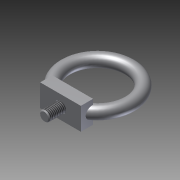
# Autodesk Inventor part: May Tec 1.71.30365_Installation ring_36.5
Saved by Autodesk Inventor 2011 SP1 (Build 150282100, 282)
## iProperties
Created: 2012-12-06
Part Number: May Tec 1.71.30365_Installation ring_36.5
Catalog Web Link: www.cadenas.de
Description: 1.71.30xxx-Installation ring
Vendor: MAYTEC
Document SubType Name: Modeling
Designer: PARTuser1
Manufacturer: MAYTEC
Density: 1 g/cm^3
Category: PARTsolutions
Company: MAYTEC
Title: May Tec 1.71.30365_Installation ring_36.5
Author: Cadenas PARTsolutions
Comments: Installation ring
PSOL_IDENT_0: {\\10.0.0.242\data_v9\23d-libs\maytec\maytec_3d\elektrozubehoer\kabelring.prj},228 {VTYP=3D},{NB=May
PSOL_IDENT_1: Tec 1.71.30365_Installation ring_36.5},{LINA=May Tec 1.71.30365_Installation ring_36.5},{NN=1.71.30
PSOL_IDENT_2: xxx},{DATE=14.09.2010 08:35:00},{GEOMDATE=28.01.2010 00:00:00},{VERSION=},{LINEID=20},{LINESUBID=-1}
PSOL_IDENT_3: ,{WBVAR=}  {NB=May Tec 1.71.30365_Installation ring_36.5},{LINA=May Tec 1.71.30365_Installation ring
PSOL_IDENT_4: _36.5},{KT=DUMMY},{PARTNR=1.71.30365},{DESCRIPTION=Kabelring},{D=36.5},{S=6.0},{XTRANS=Installation
PSOL_IDENT_5: ring}
CNS_NT: Installation ring
CNS_NB: May Tec 1.71.30365_Installation ring_36.5
CNS_NBSYN: May Tec $PARTNR._$XTRANS._$D.
CNS_LINA: May Tec 1.71.30365_Installation ring_36.5
CNS_PARTNR: 1.71.30365
CNS_DESCRIPTION: Installation ring
CNS_D: 36.5
CNS_S: 6.0
CNS_XTRANS: Installation ring
SUPPLIER: MAYTEC
ARTICLENO: May Tec 1.71.30365_Installation ring_36.5
BOMINFO: May Tec 1.71.30365_Installation ring_36.5
CREATOR: CADENAS GmbH
Autodesk Inventor part; units mm, degrees
sketch "Sketch_1" plane through (0, 0, 0) normal (1, 0, 0) x (0, 1, 0)
  line L0 (0, -50) -> (0, 50)
  circle A0 centre (15.75, 0) radius 3
  constraints: 2 end point, 1 centre point
revolve "Revolution1" add sketch "Sketch_1" angle 360 about axis through (0, 0, -50) along (0, 0, -1)
sketch "Sketch_3" plane through (0, 0, 0) normal (0, 0, 1) x (1, 0, 0)
  line L0 (-20, -23.25) -> (20, -23.25)
  line L1 (20, -23.25) -> (20, -18.25)
  line L2 (20, -18.25) -> (-20, -18.25)
  line L3 (-20, -18.25) -> (-20, -23.25)
  constraints: 8 end point
sketch "Sketch_2" plane through (0, 0, 0) normal (0, 0, 1) x (1, 0, 0)
  line L0 (-10, -18.25) -> (10, -18.25)
  line L1 (10, -18.25) -> (10, -12.25)
  line L2 (10, -12.25) -> (-10, -12.25)
  line L3 (-10, -12.25) -> (-10, -18.25)
  constraints: 8 end point
extrude "Extrusion1" add sketch "Sketch_2" along normal mid plane 11
extrude "Extrusion2" cut sketch "Sketch_3" along normal mid plane 11
sketch "Sketch_4" plane through (0, 0, 0) normal (1, 0, 0) x (0, 1, 0)
  line L0 (-50, 0) -> (50, 0)
  line L1 (-7.25, 0) -> (-7.25, -5)
  line L2 (-7.25, -5) -> (-12.25, -5)
  line L3 (-12.25, -5) -> (-14.6, -2.65)
  line L4 (-14.6, -2.65) -> (-18.25, -2.65)
  line L5 (-18.25, -2.65) -> (-18.25, 0)
  line L6 (-18.25, 0) -> (-7.25, 0)
  constraints: 14 end point
revolve "Revolution2" cut sketch "Sketch_4" angle 360 about axis through (0, -50, 0) along (0, -1, 0)
sketch "Sketch_5" plane through (0, 0, 0) normal (1, 0, 0) x (0, 1, 0)
  line L0 (-26.25, 0) -> (-12.25, 0)
  line L1 (-12.25, 0) -> (-12.25, -4.95)
  line L2 (-12.25, -4.95) -> (-14.96, -2.5)
  line L3 (-14.96, -2.5) -> (-25.7595, -2.5)
  line L4 (-25.7595, -2.5) -> (-26.25, -2.0095)
  line L5 (-26.25, -2.0095) -> (-26.25, 0)
  line L6 (-26.25, 0) -> (-12.25, 0)
  constraints: 14 end point
revolve "Revolution3" add sketch "Sketch_5" angle 360 about axis through (0, -26.25, 0) along (0, -1, 0)
thread "Thread1" size "M5x0.8" class "6g" standard "ISO Metric profile" length 10 offset 1.29
sketch "Sketch_6" plane through (0, -12.25, 0) normal (0, 1, 0) x (0, 0, -1)
  line L0 (-1.5, 0.866) -> (-1.5, -0.866)
  line L1 (-1.5, -0.866) -> (0, -1.7321)
  line L2 (0, -1.7321) -> (1.5, -0.866)
  line L3 (1.5, -0.866) -> (1.5, 0.866)
  line L4 (1.5, 0.866) -> (0, 1.7321)
  line L5 (0, 1.7321) -> (-1.5, 0.866)
  constraints: 12 end point
extrude "Extrusion3" cut sketch "Sketch_6" against normal blind 2
ref_plane "side_1_XY" through (0, -18.25, 0) normal (0, -1, 0) x (1, 0, 0)
ref_plane "side_1_YZ" through (0, -18.25, 0) normal (1, 0, 0) x (0, 0, 1)
ref_plane "side_1_ZX" through (0, -18.25, 0) normal (0, 0, 1) x (0, -1, 0)
body "Solid1"
